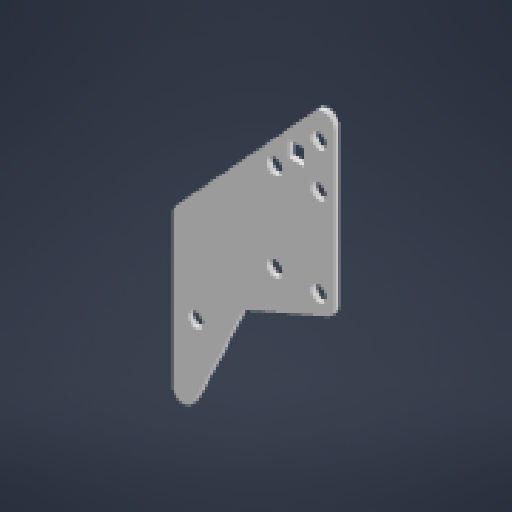
# Autodesk Inventor part: back-sled
Saved by Autodesk Inventor 2024 (Build 280153000, 153)
## iProperties
Created: 2023-04-20
Part Number: back-sled
Material: Generic
Document SubType Name: Modeling
Designer: liamt
Density: 1 g/cm^3
Appearance: Default
Author: liamt
Autodesk Inventor part; units mm, degrees
ref_plane "YZ Plane" through (0, 0, 0) normal (1, 0, 0) x (0, 1, 0)
ref_plane "XZ Plane" through (0, 0, 0) normal (0, 1, 0) x (-1, 0, 0)
ref_plane "XY Plane" through (0, 0, 0) normal (0, 0, 1) x (1, 0, 0)
sketch "Sketch1" plane through (0, 0, 0) normal (0, 0, 1) x (1, 0, 0)
  line L0 (-27.7783, -197.0642) -> (-31.3026, -204.3884)
  line L1 (-31.4232, -201.1242) -> (-27.8989, -193.8)
  line L2 (-27.8989, -193.8) -> (-23.4904, -184.6379)
  line L3 (-23.4904, -184.6379) -> (-28.7106, -195.4868)
  line L4 (-34.7466, -194.1101) -> (-34.7466, -152.2155)
  line L5 (-33.912, -150.07) -> (5.3023, -107.292)
  line L6 (10.8178, -109.4374) -> (10.8178, -153.8408)
  line L7 (8.906, -156.7537) -> (-14.4444, -166.8799)
  line L8 (-16.0666, -168.4681) -> (-23.4904, -184.6379)
  arc A0 (10.8178, -109.4374) -> (5.3023, -107.292) centre (7.6428, -109.4374) ccw
  arc A1 (8.906, -156.7537) -> (10.8178, -153.8408) centre (7.6428, -153.8408) ccw
  arc A2 (-14.4444, -166.8799) -> (-16.0666, -168.4681) centre (-13.1812, -169.7928) ccw
  arc A3 (-34.7466, -194.1101) -> (-28.7106, -195.4868) centre (-31.5716, -194.1101) ccw
  arc A4 (-33.912, -150.07) -> (-34.7466, -152.2155) centre (-31.5716, -152.2155) ccw
  circle A5 centre (6.35, -152.4) radius 2.1844
  circle A6 centre (-6.35, -152.4) radius 2.1844
  circle A7 centre (6.35, -114.3) radius 2.1844
  circle A8 centre (-6.35, -127) radius 2.1844
  circle A9 centre (-29.0224, -176.553) radius 2.0955
  line L9 (2.2749, -122.43) -> (2.2749, -121.1289)
  spline S0 degree 3 poles (2.2749, -121.1289) (2.2749, -120.7564) (2.2756, -120.3847) (2.2775, -119.644) (2.2787, -119.2745) (2.2799, -118.9051) knots 0 0 0 0 0.5 0.5 1 1 1 1
  arc A10 (1.78, -122.9249) -> (2.2749, -122.43) centre (1.78, -122.43) ccw
  arc A11 (2.2799, -118.87) -> (1.78, -118.3701) centre (1.78, -118.87) ccw
  spline S1 degree 3 poles (2.2799, -118.9051) (2.2799, -118.8934) (2.2799, -118.8817) (2.2799, -118.87) knots 0 0 0 0 1 1 1 1
  line L10 (1.78, -118.3701) -> (-1.78, -118.3701)
  arc A12 (-1.78, -118.3701) -> (-2.2799, -118.87) centre (-1.78, -118.87) ccw
  spline S2 degree 3 poles (-2.2799, -118.9051) (-2.2787, -119.2745) (-2.2775, -119.644) (-2.2756, -120.3847) (-2.2749, -120.7564) (-2.2749, -121.1289) knots 0 0 0 0 0.5 0.5 1 1 1 1
  spline S3 degree 3 poles (-2.2799, -118.87) (-2.2799, -118.8817) (-2.2799, -118.8934) (-2.2799, -118.9051) knots 0 0 0 0 1 1 1 1
  line L11 (-2.2749, -121.1289) -> (-2.2749, -122.43)
  arc A13 (-2.2749, -122.43) -> (-1.78, -122.9249) centre (-1.78, -122.43) ccw
  line L12 (-1.78, -122.9249) -> (1.78, -122.9249)
  circle A14 centre (0, -133.35) radius 2.1844
  point P0 (0, 0)
  point P1 (-34.7466, -208.031)
  dimension "d0" = 1.524
  dimension "d1" = 3.175
  dimension "d2" = 4.191
  constraints: 16 end point, 10 point on circle, 10 tangent, 7 centre point, 5 equal radius, 3 point on line, 2 parallel, 1 vertical, 2 other
  measures "d0" distance between parallel lines of L1 L0
  measures "d1" radius of A0
  measures "d2" diameter of A9
extrude "Extrusion1" add sketch "Sketch1" along normal blind 1.524
body "Solid1"
